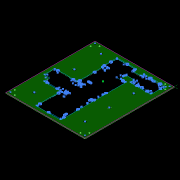
# Autodesk Inventor part: 3d_DAA_panel - Panel
Saved by Autodesk Inventor 2018 (Build 220112000, 112)
## iProperties
Created: 2024-08-29
Part Number: 3d_DAA_panel - Panel
Material: PCB
Document SubType Name: Modeling
Designer: cda1
Density: 4 g/cm^3
Appearance: PCB
Author: cda1
Autodesk Inventor part; units mm, degrees
(part 1 of 2)
ref_plane "YZ Plane" through (0, 0, 0) normal (1, 0, 0) x (0, 1, 0)
ref_plane "XZ Plane" through (0, 0, 0) normal (0, 1, 0) x (-1, 0, 0)
sketch "Boceto1" plane through (0, 0, 0) normal (0, 0, 1) x (1, 0, 0)
  circle A0 centre (-20.9021, 53.0601) radius 0.75 projected
  circle A1 centre (-25.9819, 53.0601) radius 0.75 projected
  circle A2 centre (-25.9819, 58.1399) radius 0.75 projected
  circle A3 centre (-23.442, 55.6) radius 0.7 projected
  circle A4 centre (-20.9021, 58.1399) radius 0.75 projected
  circle A5 centre (-9.192, 56.238) radius 1 projected
  circle A6 centre (-23.092, 32.962) radius 1 projected
  arc A7 (-27.742, 29.842) -> (-27.242, 29.342) centre (-27.242, 29.842) ccw projected
  line L0 (-27.242, 29.342) -> (-20.642, 29.342) projected
  arc A8 (-20.642, 29.342) -> (-20.142, 29.842) centre (-20.642, 29.842) ccw projected
  line L1 (-20.142, 29.842) -> (-20.142, 31.9) projected
  arc A9 (-19.642, 32.4) -> (-20.142, 31.9) centre (-19.642, 31.9) ccw projected
  line L2 (-19.642, 32.4) -> (12.558, 32.4) projected
  arc A10 (12.558, 32.4) -> (13.058, 32.9) centre (12.558, 32.9) ccw projected
  line L3 (13.058, 32.9) -> (13.058, 59.358) projected
  arc A11 (13.058, 59.358) -> (12.558, 59.858) centre (12.558, 59.358) ccw projected
  line L4 (12.558, 59.858) -> (-27.242, 59.858) projected
  arc A12 (-27.242, 59.858) -> (-27.742, 59.358) centre (-27.242, 59.358) ccw projected
  line L5 (-27.742, 29.842) -> (-27.742, 59.358) projected
  circle A13 centre (56.15, 55.6) radius 2 projected
  circle A14 centre (56.15, 33.6) radius 2 projected
  circle A15 centre (73, 53.6) radius 1.5 projected
  circle A16 centre (44.6, 53.6) radius 1.5 projected
  circle A17 centre (44.6, 35.6) radius 1.5 projected
  circle A18 centre (73, 35.6) radius 1.5 projected
  circle A19 centre (36.4, 32.98) radius 1 projected
  circle A20 centre (78.021, 53.178) radius 1 projected
  circle A21 centre (36.4, 56.256) radius 1 projected
  arc A22 (76.8, 32.3) -> (77.3, 32.8) centre (76.8, 32.8) ccw projected
  line L6 (77.3, 32.8) -> (77.3, 50.2) projected
  arc A23 (77.8, 50.7) -> (77.3, 50.2) centre (77.8, 50.2) ccw projected
  line L7 (77.8, 50.7) -> (79.8, 50.7) projected
  arc A24 (79.8, 50.7) -> (80.3, 51.2) centre (79.8, 51.2) ccw projected
  line L8 (80.3, 51.2) -> (80.3, 56.4) projected
  arc A25 (80.3, 56.4) -> (79.8, 56.9) centre (79.8, 56.4) ccw projected
  line L9 (79.8, 56.9) -> (58.9, 56.9) projected
  arc A26 (58.4, 57.4) -> (58.9, 56.9) centre (58.9, 57.4) ccw projected
  arc A27 (58.4, 57.4) -> (57.9, 57.9) centre (57.9, 57.4) ccw projected
  line L10 (57.9, 57.9) -> (54.4, 57.9) projected
  arc A28 (54.4, 57.9) -> (53.9, 57.4) centre (54.4, 57.4) ccw projected
  arc A29 (53.4, 56.9) -> (53.9, 57.4) centre (53.4, 57.4) ccw projected
  line L11 (53.4, 56.9) -> (39.4, 56.9) projected
  arc A30 (38.9, 57.4) -> (39.4, 56.9) centre (39.4, 57.4) ccw projected
  line L12 (38.9, 57.4) -> (38.9, 58.3) projected
  arc A31 (38.9, 58.3) -> (38.4, 58.8) centre (38.4, 58.3) ccw projected
  line L13 (38.4, 58.8) -> (34.4, 58.8) projected
  arc A32 (34.4, 58.8) -> (33.9, 58.3) centre (34.4, 58.3) ccw projected
  line L14 (33.9, 58.3) -> (33.9, 54.2) projected
  arc A33 (33.9, 54.2) -> (34.4, 53.7) centre (34.4, 54.2) ccw projected
  line L15 (34.4, 53.7) -> (36.8, 53.7) projected
  arc A34 (37.3, 53.2) -> (36.8, 53.7) centre (36.8, 53.2) ccw projected
  line L16 (37.3, 53.2) -> (37.3, 36) projected
  arc A35 (36.8, 35.5) -> (37.3, 36) centre (36.8, 36) ccw projected
  line L17 (36.8, 35.5) -> (34.4, 35.5) projected
  arc A36 (34.4, 35.5) -> (33.9, 35) centre (34.4, 35) ccw projected
  line L18 (33.9, 30.9) -> (33.9, 35) projected
  arc A37 (33.9, 30.9) -> (34.4, 30.4) centre (34.4, 30.9) ccw projected
  line L19 (34.4, 30.4) -> (38.4, 30.4) projected
  arc A38 (38.4, 30.4) -> (38.9, 30.9) centre (38.4, 30.9) ccw projected
  line L20 (38.9, 30.9) -> (38.9, 31.8) projected
  arc A39 (39.4, 32.3) -> (38.9, 31.8) centre (39.4, 31.8) ccw projected
  line L21 (39.4, 32.3) -> (53.4, 32.3) projected
  arc A40 (53.9, 31.8) -> (53.4, 32.3) centre (53.4, 31.8) ccw projected
  arc A41 (53.9, 31.8) -> (54.4, 31.3) centre (54.4, 31.8) ccw projected
  line L22 (54.4, 31.3) -> (57.9, 31.3) projected
  arc A42 (57.9, 31.3) -> (58.4, 31.8) centre (57.9, 31.8) ccw projected
  arc A43 (58.9, 32.3) -> (58.4, 31.8) centre (58.9, 31.8) ccw projected
  line L23 (58.9, 32.3) -> (76.8, 32.3) projected
  circle A44 centre (-9.825, -17.035) radius 0.37 projected
  circle A45 centre (-9.825, -15.765) radius 0.37 projected
  circle A46 centre (-11.095, -17.035) radius 0.37 projected
  circle A47 centre (-12.365, -17.035) radius 0.37 projected
  circle A48 centre (-13.635, -17.035) radius 0.37 projected
  circle A49 centre (-14.905, -15.765) radius 0.37 projected
  circle A50 centre (-16.175, -17.035) radius 0.37 projected
  circle A51 centre (-16.175, -15.765) radius 0.37 projected
  circle A52 centre (-14.905, -17.035) radius 0.37 projected
  circle A53 centre (-13.635, -15.765) radius 0.37 projected
  circle A54 centre (-12.365, -15.765) radius 0.37 projected
  circle A55 centre (-11.095, -15.765) radius 0.37 projected
  arc A56 (-20.107, 25.5) -> (-20.607, 26) centre (-20.607, 25.5) ccw projected
  line L24 (-25.5, 26) -> (-20.607, 26) projected
  arc A57 (-25.5, 26) -> (-26, 25.5) centre (-25.5, 25.5) ccw projected
  line L25 (-26, -28) -> (-26, 25.5) projected
  arc A58 (-26, -28) -> (-25.5, -28.5) centre (-25.5, -28) ccw projected
  line L26 (-16, -28.5) -> (-25.5, -28.5) projected
  arc A59 (-16, -28.5) -> (-15.5, -28) centre (-16, -28) ccw projected
  line L27 (-15.5, -26.5) -> (-15.5, -28) projected
  arc A60 (-15, -26) -> (-15.5, -26.5) centre (-15, -26.5) ccw projected
  line L28 (25.5, -26) -> (-15, -26) projected
  arc A61 (25.5, -26) -> (26, -25.5) centre (25.5, -25.5) ccw projected
  line L29 (26, 22) -> (26, -25.5) projected
  arc A62 (26, 22) -> (25, 23) centre (25, 22) ccw projected
  line L30 (25, 23) -> (-19.607, 23) projected
  arc A63 (-20.107, 23.5) -> (-19.607, 23) centre (-19.607, 23.5) ccw projected
  line L31 (-20.107, 23.5) -> (-20.107, 25.5) projected
  arc A64 (-15.5, -32.942) -> (-16, -32.442) centre (-16, -32.942) ccw projected
  line L32 (-16, -32.442) -> (-22.3, -32.442) projected
  arc A65 (-22.3, -32.442) -> (-22.8, -32.942) centre (-22.3, -32.942) ccw projected
  line L33 (-22.8, -32.942) -> (-22.8, -62.458) projected
  arc A66 (-22.8, -62.458) -> (-22.3, -62.958) centre (-22.3, -62.458) ccw projected
  line L34 (-22.3, -62.958) -> (-16, -62.958) projected
  arc A67 (-16, -62.958) -> (-15.5, -62.458) centre (-16, -62.458) ccw projected
  line L35 (-15.5, -62.458) -> (-15.5, -60.4) projected
  arc A68 (-15, -59.9) -> (-15.5, -60.4) centre (-15, -60.4) ccw projected
  line L36 (-15, -59.9) -> (25.5, -59.9) projected
  arc A69 (25.5, -59.9) -> (26, -59.4) centre (25.5, -59.4) ccw projected
  line L37 (26, -36) -> (26, -59.4) projected
  arc A70 (26, -36) -> (25.5, -35.5) centre (25.5, -36) ccw projected
  line L38 (25.5, -35.5) -> (-15, -35.5) projected
  arc A71 (-15.5, -35) -> (-15, -35.5) centre (-15, -35) ccw projected
  line L39 (-15.5, -35) -> (-15.5, -32.942) projected
  circle A72 centre (22.935, -52.24) radius 0.37 projected
  circle A73 centre (21.665, -52.24) radius 0.37 projected
  circle A74 centre (21.665, -50.97) radius 0.37 projected
  circle A75 centre (21.665, -49.7) radius 0.37 projected
  circle A76 centre (22.935, -48.43) radius 0.37 projected
  circle A77 centre (21.665, -47.16) radius 0.37 projected
  circle A78 centre (22.935, -47.16) radius 0.37 projected
  circle A79 centre (21.665, -48.43) radius 0.37 projected
  circle A80 centre (22.935, -49.7) radius 0.37 projected
  circle A81 centre (22.935, -50.97) radius 0.37 projected
  circle A82 centre (-19.1, -36.062) radius 1 projected
  circle A83 centre (-19.1, -59.338) radius 1 projected
  circle A84 centre (-47.178, -49.615) radius 0.65 projected
  circle A85 centre (-50.172, -48.173) radius 0.65 projected
  circle A86 centre (-48.1, -45.575) radius 0.65 projected
  circle A87 centre (-44.129, -48.182) radius 0.65 projected
  circle A88 centre (-46.241, -51.242) radius 0.65 projected
  circle A89 centre (-49.959, -51.242) radius 0.65 projected
  circle A90 centre (-52.071, -48.182) radius 0.65 projected
  circle A91 centre (-50.752, -44.706) radius 0.65 projected
  circle A92 centre (-47.143, -43.816) radius 0.65 projected
  circle A93 centre (-44.36, -46.282) radius 0.65 projected
  circle A94 centre (-42.297, -46.781) radius 0.65 projected
  circle A95 centre (-42.865, -50.367) radius 0.65 projected
  circle A96 centre (-45.433, -52.935) radius 0.65 projected
  circle A97 centre (-49.019, -53.503) radius 0.65 projected
  circle A98 centre (-52.254, -51.854) radius 0.65 projected
  circle A99 centre (-53.903, -48.619) radius 0.65 projected
  circle A100 centre (-53.335, -45.033) radius 0.65 projected
  circle A101 centre (-50.767, -42.465) radius 0.65 projected
  circle A102 centre (-47.181, -41.897) radius 0.65 projected
  circle A103 centre (-43.946, -43.546) radius 0.65 projected
  circle A104 centre (-41.884, -52.328) radius 0.65 projected
  circle A105 centre (-44.622, -54.626) radius 0.65 projected
  circle A106 centre (-48.1, -55.45) radius 0.65 projected
  circle A107 centre (-51.578, -54.626) radius 0.65 projected
  circle A108 centre (-54.316, -52.328) radius 0.65 projected
  circle A109 centre (-55.732, -49.046) radius 0.65 projected
  circle A110 centre (-55.524, -45.477) radius 0.65 projected
  circle A111 centre (-53.737, -42.382) radius 0.65 projected
  circle A112 centre (-50.751, -40.417) radius 0.65 projected
  circle A113 centre (-47.2, -40.002) radius 0.65 projected
  circle A114 centre (-43.841, -41.225) radius 0.65 projected
  circle A115 centre (-41.388, -43.825) radius 0.65 projected
  circle A116 centre (-40.363, -47.249) radius 0.65 projected
  circle A117 centre (-56.355, -55.955) radius 0.65 projected
  circle A118 centre (-48.1, -47.7) radius 0.65 projected
  circle A119 centre (-39.845, -39.445) radius 0.65 projected
  circle A120 centre (-56.355, -39.445) radius 0.65 projected
  circle A121 centre (-39.845, -55.955) radius 0.65 projected
  circle A122 centre (-40.468, -49.046) radius 0.65 projected
  circle A123 centre (-40.676, -45.477) radius 0.65 projected
  circle A124 centre (-42.463, -42.382) radius 0.65 projected
  circle A125 centre (-45.449, -40.417) radius 0.65 projected
  circle A126 centre (-49, -40.002) radius 0.65 projected
  circle A127 centre (-52.359, -41.225) radius 0.65 projected
  circle A128 centre (-54.812, -43.825) radius 0.65 projected
  circle A129 centre (-55.837, -47.249) radius 0.65 projected
  circle A130 centre (-55.216, -50.77) radius 0.65 projected
  circle A131 centre (-53.082, -53.637) radius 0.65 projected
  circle A132 centre (-49.887, -55.241) radius 0.65 projected
  circle A133 centre (-46.313, -55.241) radius 0.65 projected
  circle A134 centre (-43.118, -53.637) radius 0.65 projected
  circle A135 centre (-40.984, -50.77) radius 0.65 projected
  circle A136 centre (-45.433, -42.465) radius 0.65 projected
  circle A137 centre (-49.019, -41.897) radius 0.65 projected
  circle A138 centre (-52.254, -43.546) radius 0.65 projected
  circle A139 centre (-53.903, -46.781) radius 0.65 projected
  circle A140 centre (-53.335, -50.367) radius 0.65 projected
  circle A141 centre (-50.767, -52.935) radius 0.65 projected
  circle A142 centre (-47.181, -53.503) radius 0.65 projected
  circle A143 centre (-43.946, -51.854) radius 0.65 projected
  circle A144 centre (-42.297, -48.619) radius 0.65 projected
  circle A145 centre (-42.865, -45.033) radius 0.65 projected
  circle A146 centre (-45.448, -44.706) radius 0.65 projected
  circle A147 centre (-49.057, -43.816) radius 0.65 projected
  circle A148 centre (-51.84, -46.282) radius 0.65 projected
  circle A149 centre (-51.392, -49.972) radius 0.65 projected
  circle A150 centre (-48.1, -51.7) radius 0.65 projected
  circle A151 centre (-44.808, -49.972) radius 0.65 projected
  circle A152 centre (-46.439, -46.375) radius 0.65 projected
  circle A153 centre (-49.761, -46.375) radius 0.65 projected
  circle A154 centre (-49.022, -49.615) radius 0.65 projected
  circle A155 centre (-46.028, -48.173) radius 0.65 projected
  arc A156 (-77.3, -49.2) -> (-75.3, -51.2) centre (-75.3, -49.2) ccw projected
  line L40 (-75.3, -51.2) -> (-71.048, -51.2) projected
  arc A157 (-65.048, -57.2) -> (-71.048, -51.2) centre (-71.048, -57.2) ccw projected
  line L41 (-65.048, -57.2) -> (-65.048, -62.7) projected
  arc A158 (-65.048, -62.7) -> (-63.048, -64.7) centre (-63.048, -62.7) ccw projected
  line L42 (-30.8, -64.7) -> (-63.048, -64.7) projected
  arc A159 (-30.8, -64.7) -> (-30.3, -64.2) centre (-30.8, -64.2) ccw projected
  line L43 (-30.3, -64.2) -> (-30.3, -31.2) projected
  arc A160 (-30.3, -31.2) -> (-30.8, -30.7) centre (-30.8, -31.2) ccw projected
  line L44 (-76.8, -30.7) -> (-30.8, -30.7) projected
  arc A161 (-76.8, -30.7) -> (-77.3, -31.2) centre (-76.8, -31.2) ccw projected
  line L45 (-77.3, -31.2) -> (-77.3, -49.2) projected
  circle A162 centre (-67.2, -34.022) radius 1 projected
  circle A163 centre (-36.6, -34.022) radius 1 projected
  circle A164 centre (-36.6, -61.378) radius 1 projected
  arc A165 (-25.5, -66.1) -> (-26, -66.6) centre (-25.5, -66.6) ccw projected
  line L46 (-26, -120.1) -> (-26, -66.6) projected
  arc A166 (-26, -120.1) -> (-25.5, -120.6) centre (-25.5, -120.1) ccw projected
  line L47 (25.5, -120.6) -> (-25.5, -120.6) projected
  arc A167 (25.5, -120.6) -> (26, -120.1) centre (25.5, -120.1) ccw projected
  line L48 (26, -73.9) -> (26, -120.1) projected
  arc A168 (26, -73.9) -> (25.5, -73.4) centre (25.5, -73.9) ccw projected
  line L49 (25.5, -73.4) -> (-15, -73.4) projected
  arc A169 (-15.5, -72.9) -> (-15, -73.4) centre (-15, -72.9) ccw projected
  line L50 (-15.5, -72.9) -> (-15.5, -66.6) projected
  arc A170 (-15.5, -66.6) -> (-16, -66.1) centre (-16, -66.6) ccw projected
  line L51 (-25.5, -66.1) -> (-16, -66.1) projected
  circle A171 centre (23.035, -108.94) radius 0.37 projected
  circle A172 centre (21.765, -108.94) radius 0.37 projected
  circle A173 centre (21.765, -107.67) radius 0.37 projected
  circle A174 centre (21.765, -106.4) radius 0.37 projected
  circle A175 centre (21.765, -105.13) radius 0.37 projected
  circle A176 centre (23.035, -103.86) radius 0.37 projected
  circle A177 centre (21.765, -103.86) radius 0.37 projected
  circle A178 centre (23.035, -105.13) radius 0.37 projected
  circle A179 centre (23.035, -106.4) radius 0.37 projected
  circle A180 centre (23.035, -107.67) radius 0.37 projected
  line L52 (-87.3, 69.858) -> (90.3, 69.858)
  line L53 (90.3, 69.858) -> (90.3, -130.6)
  line L54 (90.3, -130.6) -> (-87.3, -130.6)
  line L55 (-87.3, -130.6) -> (-87.3, 69.858)
  line L56 (14.1664, 40.6) -> (14.1664, 52) projected
  line L57 (14.1664, 52) -> (13.0584, 52) projected
  line L58 (13.0584, 40.6) -> (13.0584, 52) projected
  line L59 (14.1664, 40.6) -> (13.0584, 40.6) projected
  line L60 (14.1664, 40.6) -> (14.1664, 52) projected
  line L61 (18.9048, 40.6) -> (14.1664, 40.6) projected
  line L62 (18.9048, 40.6) -> (18.9048, 52) projected
  line L63 (18.9048, 52) -> (14.1664, 52) projected
  line L64 (18.9048, 40.6) -> (18.9048, 52) projected
  line L65 (27.24, 40.6) -> (18.9048, 40.6) projected
  line L66 (27.24, 40.6) -> (27.24, 52) projected
  line L67 (27.24, 52) -> (18.9048, 52) projected
  line L68 (27.24, 40.6) -> (27.24, 52) projected
  line L69 (36.2006, 40.6) -> (27.24, 40.6) projected
  line L70 (36.2006, 40.6) -> (36.2006, 52) projected
  line L71 (36.2006, 52) -> (27.24, 52) projected
  line L72 (36.2006, 40.6) -> (36.2006, 52) projected
  line L73 (37.3, 40.6) -> (36.2006, 40.6) projected
  line L74 (37.3, 40.6) -> (37.3, 52) projected
  line L75 (37.3, 52) -> (36.2006, 52) projected
  line L76 (-17.807, 32.1945) -> (7.393, 32.1945) projected
  line L77 (7.393, 32.4003) -> (7.393, 32.1945) projected
  line L78 (-17.807, 32.4003) -> (7.393, 32.4003) projected
  line L79 (-17.807, 32.1945) -> (-17.807, 32.4003) projected
  line L80 (-17.807, 32.1945) -> (7.393, 32.1945) projected
  line L81 (-17.807, 30.0192) -> (-17.807, 32.1945) projected
  line L82 (-17.807, 30.0192) -> (7.393, 30.0192) projected
  line L83 (7.393, 32.1945) -> (7.393, 30.0192) projected
  line L84 (-17.807, 30.0192) -> (7.393, 30.0192) projected
  line L85 (-17.807, 24.6786) -> (-17.807, 30.0192) projected
  line L86 (-17.807, 24.6786) -> (7.393, 24.6786) projected
  line L87 (7.393, 30.0192) -> (7.393, 24.6786) projected
  line L88 (-17.807, 24.3258) -> (7.393, 24.3258) projected
  line L89 (-17.807, 23.636) -> (-17.807, 24.3258) projected
  line L90 (-17.807, 23.636) -> (7.393, 23.636) projected
  line L91 (7.393, 24.3258) -> (7.393, 23.636) projected
  line L92 (-17.807, 24.6786) -> (7.393, 24.6786) projected
  line L93 (-17.807, 24.3258) -> (-17.807, 24.6786) projected
  line L94 (-17.807, 24.3258) -> (7.393, 24.3258) projected
  line L95 (7.393, 24.6786) -> (7.393, 24.3258) projected
  line L96 (-17.807, 23.636) -> (7.393, 23.636) projected
  line L97 (-17.807, 23) -> (-17.807, 23.636) projected
  line L98 (7.393, 23) -> (-17.807, 23) projected
  line L99 (7.393, 23.636) -> (7.393, 23) projected
  line L100 (24.5, -26.636) -> (-13, -26.636) projected
  line L101 (24.5, -26) -> (24.5, -26.636) projected
  line L102 (-13, -26) -> (24.5, -26) projected
  line L103 (-13, -26.636) -> (-13, -26) projected
  line L104 (24.5, -27.3258) -> (-13, -27.3258) projected
  line L105 (24.5, -26.636) -> (24.5, -27.3258) projected
  line L106 (24.5, -26.636) -> (-13, -26.636) projected
  line L107 (-13, -27.3258) -> (-13, -26.636) projected
  line L108 (24.5, -27.6786) -> (-13, -27.6786) projected
  line L109 (24.5, -27.3258) -> (24.5, -27.6786) projected
  line L110 (24.5, -27.3258) -> (-13, -27.3258) projected
  line L111 (-13, -27.6786) -> (-13, -27.3258) projected
  line L112 (24.5, -33.0192) -> (-13, -33.0192) projected
  line L113 (24.5, -27.6786) -> (24.5, -33.0192) projected
  line L114 (24.5, -27.6786) -> (-13, -27.6786) projected
  line L115 (-13, -33.0192) -> (-13, -27.6786) projected
  line L116 (24.5, -35.1945) -> (-13, -35.1945) projected
  line L117 (24.5, -33.0192) -> (24.5, -35.1945) projected
  line L118 (24.5, -33.0192) -> (-13, -33.0192) projected
  line L119 (-13, -35.1945) -> (-13, -33.0192) projected
  line L120 (24.5, -35.1945) -> (-13, -35.1945) projected
  line L121 (-13, -35.5003) -> (-13, -35.1945) projected
  line L122 (24.5, -35.5003) -> (-13, -35.5003) projected
  line L123 (24.5, -35.1945) -> (24.5, -35.5003) projected
  line L124 (-24.064, -38) -> (-24.064, -59.3) projected
  line L125 (-24.064, -59.3) -> (-22.8, -59.3) projected
  line L126 (-22.8, -38) -> (-22.8, -59.3) projected
  line L127 (-24.064, -38) -> (-22.8, -38) projected
  line L128 (-24.064, -38) -> (-24.064, -59.3) projected
  line L129 (-28.2863, -38) -> (-24.064, -38) projected
  line L130 (-28.2863, -38) -> (-28.2863, -59.3) projected
  line L131 (-28.2863, -59.3) -> (-24.064, -59.3) projected
  line L132 (-28.2863, -38) -> (-28.2863, -59.3) projected
  line L133 (-30.2998, -38) -> (-28.2863, -38) projected
  line L134 (-30.2998, -38) -> (-30.2998, -59.3) projected
  line L135 (-30.2998, -59.3) -> (-28.2863, -59.3) projected
  line L136 (24.5, -72.6558) -> (-13, -72.6558) projected
  line L137 (-13, -72.6558) -> (-13, -73.4) projected
  line L138 (24.5, -73.4) -> (-13, -73.4) projected
  line L139 (24.5, -72.6558) -> (24.5, -73.4) projected
  line L140 (24.5, -72.6558) -> (-13, -72.6558) projected
  line L141 (24.5, -71.0155) -> (24.5, -72.6558) projected
  line L142 (24.5, -71.0155) -> (-13, -71.0155) projected
  line L143 (-13, -71.0155) -> (-13, -72.6558) projected
  line L144 (24.5, -71.0155) -> (-13, -71.0155) projected
  line L145 (24.5, -61.4174) -> (24.5, -71.0155) projected
  line L146 (24.5, -61.4174) -> (-13, -61.4174) projected
  line L147 (-13, -61.4174) -> (-13, -71.0155) projected
  line L148 (24.5, -61.4174) -> (-13, -61.4174) projected
  line L149 (24.5, -61.3135) -> (24.5, -61.4174) projected
  line L150 (24.5, -61.3135) -> (-13, -61.3135) projected
  line L151 (-13, -61.3135) -> (-13, -61.4174) projected
  line L152 (24.5, -61.3135) -> (-13, -61.3135) projected
  line L153 (24.5, -60.0991) -> (24.5, -61.3135) projected
  line L154 (24.5, -60.0991) -> (-13, -60.0991) projected
  line L155 (-13, -60.0991) -> (-13, -61.3135) projected
  line L156 (24.5, -60.0991) -> (-13, -60.0991) projected
  line L157 (24.5, -59.8978) -> (24.5, -60.0991) projected
  line L158 (24.5, -59.8978) -> (-13, -59.8978) projected
  line L159 (-13, -59.8978) -> (-13, -60.0991) projected
  line L160 (-79.3, -29.7) -> (-79.3, -52.2)
  arc A181 (-67.048, -57.2) -> (-71.048, -53.2) centre (-71.048, -57.2) ccw
  line L161 (-71.048, -53.2) -> (-78.3, -53.2)
  line L162 (-67.048, -57.2) -> (-67.048, -65.7)
  line L163 (15.058, 25) -> (15.058, 34.6)
  line L164 (15.058, 36.6) -> (31.9, 36.6)
  line L165 (31.9, 36.6) -> (31.9, 29.4)
  line L166 (79.3, 29.4) -> (79.3, 47.7)
  line L167 (80.3, 48.7) -> (81.3, 48.7)
  line L168 (82.3, 49.7) -> (82.3, 59.8)
  line L169 (31.9, 59.8) -> (31.9, 56)
  line L170 (31.9, 56) -> (15.058, 56)
  line L171 (15.058, 58) -> (15.058, 60.858)
  line L172 (-28.742, 27.342) -> (-28, 27.342)
  arc A182 (-78.3, -28.7) -> (-79.3, -29.7) centre (-78.3, -29.7) ccw
  arc A183 (-79.3, -52.2) -> (-78.3, -53.2) centre (-78.3, -52.2) ccw
  arc A184 (-67.048, -65.7) -> (-66.048, -66.7) centre (-66.048, -65.7) ccw
  arc A185 (-28, -121.6) -> (-27, -122.6) centre (-27, -121.6) ccw
  arc A186 (27, -122.6) -> (28, -121.6) centre (27, -121.6) ccw
  arc A187 (28, 24) -> (27, 25) centre (27, 24) ccw
  arc A188 (31.9, 29.4) -> (32.9, 28.4) centre (32.9, 29.4) ccw
  arc A189 (78.3, 28.4) -> (79.3, 29.4) centre (78.3, 29.4) ccw
  arc A190 (80.3, 48.7) -> (79.3, 47.7) centre (80.3, 47.7) ccw
  arc A191 (81.3, 48.7) -> (82.3, 49.7) centre (81.3, 49.7) ccw
  arc A192 (82.3, 59.8) -> (81.3, 60.8) centre (81.3, 59.8) ccw
  arc A193 (32.9, 60.8) -> (31.9, 59.8) centre (32.9, 59.8) ccw
  arc A194 (15.058, 60.858) -> (14.058, 61.858) centre (14.058, 60.858) ccw
  arc A195 (-28.742, 61.858) -> (-29.742, 60.858) centre (-28.742, 60.858) ccw
  arc A196 (-29.742, 28.342) -> (-28.742, 27.342) centre (-28.742, 28.342) ccw
  line L173 (-20.3, -28.5) -> (-18.3, -28.5)
  line L174 (-18.3, -28.5) -> (-18.3, -32.442)
  line L175 (-18.3, -32.442) -> (-20.3, -32.442)
  line L176 (-20.3, -32.442) -> (-20.3, -28.5)
  line L177 (-20.3, -62.958) -> (-18.3, -62.958)
  line L178 (-18.3, -62.958) -> (-18.3, -66.1)
  line L179 (-18.3, -66.1) -> (-20.3, -66.1)
  line L180 (-20.3, -66.1) -> (-20.3, -62.958)
  line L181 (-60.048, -64.7) -> (-60.048, -66.7)
  line L182 (-58.048, -64.7) -> (-58.048, -66.7)
  line L183 (-37.3, -64.7) -> (-37.3, -66.7)
  line L184 (-35.3, -64.7) -> (-35.3, -66.7)
  line L185 (-72.3, -28.7) -> (-72.3, -30.7)
  line L186 (-70.3, -28.7) -> (-70.3, -30.7)
  line L187 (-37.3, -28.7) -> (-37.3, -30.7)
  line L188 (-35.3, -28.7) -> (-35.3, -30.7)
  line L189 (-29.742, 31.342) -> (-27.742, 31.342)
  line L190 (-29.742, 33.342) -> (-27.742, 33.342)
  line L191 (-29.742, 47.858) -> (-27.742, 47.858)
  line L192 (-27.742, 45.858) -> (-29.742, 45.858)
  line L193 (15.058, 36.6) -> (13.058, 36.6)
  line L194 (15.058, 34.6) -> (13.058, 34.6)
  line L195 (15.058, 56) -> (13.058, 56)
  line L196 (15.058, 58) -> (13.058, 58)
  line L197 (48.7, 56.9) -> (48.7, 60.8)
  line L198 (46.7, 56.9) -> (46.7, 60.8)
  line L199 (68.7, 56.9) -> (68.7, 60.8)
  line L200 (70.7, 56.9) -> (70.7, 60.8)
  line L201 (70.7, 32.3) -> (70.7, 28.4)
  line L202 (68.7, 32.3) -> (68.7, 28.4)
  line L203 (48.7, 32.3) -> (48.7, 28.4)
  line L204 (46.7, 32.3) -> (46.7, 28.4)
  line L205 (20, 25) -> (20, 23)
  line L206 (22, 25) -> (22, 23)
  line L207 (-26, 9.6) -> (-28, 9.6)
  line L208 (-26, 7.6) -> (-28, 7.6)
  line L209 (-26, -25.5) -> (-28, -25.5)
  line L210 (-26, -23.5) -> (-28, -23.5)
  line L211 (26, -21) -> (28, -21)
  line L212 (26, -19) -> (28, -19)
  line L213 (26, -45.7) -> (28, -45.7)
  line L214 (26, -49.7) -> (28, -49.7)
  line L215 (-28, -71.1) -> (-26, -71.1)
  line L216 (-28, -73.1) -> (-26, -73.1)
  line L217 (-28, -115.6) -> (-26, -115.6)
  line L218 (-28, -113.6) -> (-26, -113.6)
  line L219 (-1, -120.6) -> (-1, -122.6)
  line L220 (1, -120.6) -> (1, -122.6)
  line L221 (26, -81.8) -> (28, -81.8)
  line L222 (26, -83.8) -> (28, -83.8)
  line L223 (26, -113.6) -> (28, -113.6)
  line L224 (26, -115.6) -> (28, -115.6)
  line L225 (20, 23) -> (22, 23)
  line L226 (13.058, 34.6) -> (13.058, 36.6)
  line L227 (46.7, 32.3) -> (48.7, 32.3)
  line L228 (68.7, 32.3) -> (70.7, 32.3)
  line L229 (68.7, 56.9) -> (70.7, 56.9)
  line L230 (48.7, 56.9) -> (46.7, 56.9)
  line L231 (13.058, 58) -> (13.058, 56)
  line L232 (-27.742, 47.858) -> (-27.742, 45.858)
  line L233 (-27.742, 33.342) -> (-27.742, 31.342)
  line L234 (-26, 9.6) -> (-26, 7.6)
  line L235 (-26, -23.5) -> (-26, -25.5)
  line L236 (-35.3, -30.7) -> (-37.3, -30.7)
  line L237 (-72.3, -30.7) -> (-70.3, -30.7)
  line L238 (-60.048, -64.7) -> (-58.048, -64.7)
  line L239 (-37.3, -64.7) -> (-35.3, -64.7)
  line L240 (-26, -71.1) -> (-26, -73.1)
  line L241 (-26, -113.6) -> (-26, -115.6)
  line L242 (-1, -120.6) -> (1, -120.6)
  line L243 (26, -115.6) -> (26, -113.6)
  line L244 (26, -81.8) -> (26, -83.8)
  line L245 (26, -45.7) -> (26, -49.7)
  line L246 (26, -19) -> (26, -21)
  line L247 (-72.3, -28.7) -> (-78.3, -28.7)
  line L248 (-28, -28.7) -> (-35.3, -28.7)
  line L249 (-37.3, -28.7) -> (-70.3, -28.7)
  line L250 (-66.048, -66.7) -> (-60.048, -66.7)
  line L251 (-58.048, -66.7) -> (-37.3, -66.7)
  line L252 (-35.3, -66.7) -> (-28, -66.7)
  line L253 (-28, -66.7) -> (-28, -71.1)
  line L254 (-28, -73.1) -> (-28, -113.6)
  line L255 (-28, -115.6) -> (-28, -121.6)
  line L256 (-27, -122.6) -> (-1, -122.6)
  line L257 (1, -122.6) -> (27, -122.6)
  line L258 (28, -121.6) -> (28, -115.6)
  line L259 (28, -113.6) -> (28, -83.8)
  line L260 (28, -81.8) -> (28, -49.7)
  line L261 (28, -45.7) -> (28, -21)
  line L262 (28, -19) -> (28, 24)
  line L263 (27, 25) -> (22, 25)
  line L264 (20, 25) -> (15.058, 25)
  line L265 (32.9, 28.4) -> (46.7, 28.4)
  line L266 (48.7, 28.4) -> (68.7, 28.4)
  line L267 (70.7, 28.4) -> (78.3, 28.4)
  line L268 (81.3, 60.8) -> (70.7, 60.8)
  line L269 (68.7, 60.8) -> (48.7, 60.8)
  line L270 (46.7, 60.8) -> (32.9, 60.8)
  line L271 (-29.742, 60.858) -> (-29.742, 47.858)
  line L272 (-29.742, 45.858) -> (-29.742, 33.342)
  line L273 (-29.742, 31.342) -> (-29.742, 28.342)
  line L274 (-28, 27.342) -> (-28, 9.6)
  line L275 (-28, 7.6) -> (-28, -23.5)
  line L276 (-28, -25.5) -> (-28, -28.7)
  line L277 (26, -47.7) -> (28, -47.7) construction
  line L278 (-6.6, 61.858) -> (-6.6, 59.858)
  line L279 (-4.6, 61.858) -> (-4.6, 59.858)
  line L280 (-4.6, 59.858) -> (-6.6, 59.858)
  line L281 (14.058, 61.858) -> (-4.6, 61.858)
  line L282 (-6.6, 61.858) -> (-28.742, 61.858)
  point P0 (0, 0)
  dimension "d0" = 10
  dimension "d1" = 10
  dimension "d2" = 10
  dimension "d3" = 10
  dimension "d4" = 2
  dimension "d6" = 2
  dimension "d10" = 2
  dimension "d11" = 2
  dimension "d12" = 2
  dimension "d14" = 2
  dimension "d19" = 2
  dimension "d21" = 4
  dimension "d22" = 4
  dimension "d23" = 2
  dimension "d24" = 2
  dimension "d25" = 2
  dimension "d28" = 1
  dimension "d29" = 1
  dimension "d30" = 2
  dimension "d31" = 2
  dimension "d32" = 2.5
  dimension "d33" = 2
  dimension "d34" = 2
  dimension "d35" = 2
  dimension "d36" = 2
  dimension "d37" = 2
  dimension "d38" = 2
  dimension "d39" = 2
  dimension "d40" = 2
  dimension "d42" = 2
  dimension "d43" = 2
  dimension "d44" = 2
  dimension "d45" = 2
  dimension "d46" = 6.6
  dimension "d47" = 12.8
  dimension "d48" = 12.8
  dimension "d49" = 9.6
  dimension "d50" = 2
  dimension "d51" = 12
  dimension "d52" = 5
  dimension "d53" = 5
  dimension "d54" = 5
  dimension "d55" = 5
  dimension "d56" = 2
  dimension "d57" = 4
  dimension "d58" = 2
  dimension "d59" = 16.4
  dimension "d60" = 2
  dimension "d62" = 3
  dimension "d63" = 2
  dimension "d64" = 5
  dimension "d65" = 4
  dimension "d69" = 2
  dimension "d70" = 2
  dimension "d71" = 2
  dimension "d72" = 2
  dimension "d73" = 2
  dimension "d74" = 5
  dimension "d75" = 5
  dimension "d76" = 5
  dimension "d77" = 8.4
  dimension "d79" = 2
  dimension "d80" = 2
  dimension "d81" = 2
  constraints: 254 end point, 170 perpendicular, 63 tangent, 51 point on line, 32 point on circle, 18 collinear, 16 centre point, 16 parallel, 13 equal radius, 11 horizontal, 3 vertical, 1 coincident, 1 midpoint, 1 vertical alignment
  measures "d0" distance between parallel lines of L54 L47
  measures "d1" distance between parallel lines of L52 L4
  measures "d2" distance between parallel lines of L55 L45
  measures "d3" distance between parallel lines of L53 L8
  measures "d4" distance between parallel lines of L162 L41
  measures "d6" distance between parallel lines of L160 L45
  measures "d10" distance between parallel lines of L0 L172
  measures "d11" distance between parallel lines of L163 L3
  measures "d12" distance between parallel lines of L171 L3
  measures "d14" distance between parallel lines of L165 L18
  measures "d19" distance between parallel lines of L14 L169
  measures "d21" distance between parallel lines of L67 L170
  measures "d22" distance between parallel lines of L164 L65
  measures "d23" distance between parallel lines of L166 L6
  measures "d24" distance between parallel lines of L168 L8
  measures "d25" distance between parallel lines of L167 L7
  measures "d28" radius of A182
  measures "d29" radius of A189
  measures "d30" distance between parallel lines of L176 L174
  measures "d31" distance between parallel lines of L178 L180
  measures "d32" distance between parallel lines of L33 L176
  measures "d33" distance between parallel lines of L182 L181
  measures "d34" distance between parallel lines of L184 L183
  measures "d35" distance between parallel lines of L185 L186
  measures "d36" distance between parallel lines of L187 L188
  measures "d37" distance between parallel lines of L189 L190
  measures "d38" distance between parallel lines of L191 L192
  measures "d39" distance between parallel lines of L194 L193
  measures "d40" distance between parallel lines of L195 L196
  measures "d42" distance between parallel lines of L198 L197
  measures "d43" distance between parallel lines of L204 L203
  measures "d44" distance between parallel lines of L202 L201
  measures "d45" distance between parallel lines of L200 L199
  measures "d46" distance between parallel lines of L6 L201
  measures "d47" distance between parallel lines of L18 L204
  measures "d48" distance between parallel lines of L14 L198
  measures "d49" distance between parallel lines of L8 L200
  measures "d50" distance between parallel lines of L0 L189
  measures "d51" distance between parallel lines of L4 L191
  measures "d52" distance from line of L185 L45.start
  measures "d53" distance from line of L188 L43.end
  measures "d54" distance from line of L184 L43.start
  measures "d55" distance from line of L41.end L181
  measures "d56" distance between parallel lines of L206 L205
  measures "d57" distance between parallel lines of L206 L29
  measures "d58" distance between parallel lines of L208 L207
  measures "d59" distance between parallel lines of L24 L207
  measures "d60" distance between parallel lines of L209 L210
  measures "d62" distance from line of L209 L26.end
  measures "d63" distance between parallel lines of L211 L212
  measures "d64" distance between parallel lines of L211 L28
  measures "d65" distance between parallel lines of L213 L214
  measures "d69" distance between parallel lines of L224 L223
  measures "d70" distance between parallel lines of L222 L221
  measures "d71" distance between parallel lines of L220 L219
  measures "d72" distance between parallel lines of L218 L217
  measures "d73" distance between parallel lines of L216 L215
  measures "d74" distance between parallel lines of L51 L215
  measures "d75" distance between parallel lines of L47 L217
  measures "d76" distance between parallel lines of L47 L224
  measures "d77" distance between parallel lines of L49 L221
  measures "d79" distance from line of L247 L44.start
  measures "d80" distance from line of L42.end L250
  measures "d81" distance between parallel lines of L46 L253
extrude "Extrusión1" add sketch "Boceto1" against normal blind 1.742 contours L26 L174 L32 L176 | L34 L178 L51 L180 | L52 L53 L54 L55
sketch "Boceto2" plane through (0, 0, 0) normal (0, 0, 1) x (1, 0, 0)
  line L0 (-26, 7.6) -> (-26, 9.6) construction
  line L1 (-26, 9.6) -> (-28, 9.6) construction
  line L2 (-28, 9.6) -> (-28, 27.342) construction
  line L3 (-28, 27.342) -> (-28.742, 27.342) construction
  arc A0 (-29.742, 28.342) -> (-28.742, 27.342) centre (-28.742, 28.342) ccw construction
  line L4 (-29.742, 28.342) -> (-29.742, 31.342) construction
  line L5 (-29.742, 31.342) -> (-27.742, 31.342) construction
  line L6 (-27.742, 31.342) -> (-27.742, 33.342) construction
  line L7 (-27.742, 33.342) -> (-29.742, 33.342) construction
  line L8 (-29.742, 33.342) -> (-29.742, 45.858) construction
  line L9 (-29.742, 45.858) -> (-27.742, 45.858) construction
  line L10 (-27.742, 45.858) -> (-27.742, 47.858) construction
  line L11 (-27.742, 47.858) -> (-29.742, 47.858) construction
  line L12 (-29.742, 47.858) -> (-29.742, 60.858) construction
  arc A1 (-28.742, 61.858) -> (-29.742, 60.858) centre (-28.742, 60.858) ccw construction
  line L13 (-4.6, 61.858) -> (14.058, 61.858) construction
  arc A2 (15.058, 60.858) -> (14.058, 61.858) centre (14.058, 60.858) ccw construction
  line L14 (15.058, 60.858) -> (15.058, 58) construction
  line L15 (15.058, 58) -> (13.058, 58) construction
  line L16 (13.058, 36.6) -> (13.058, 34.6) construction
  line L17 (13.058, 56) -> (31.9, 56) construction
  line L18 (31.9, 56) -> (31.9, 59.8) construction
  arc A3 (32.9, 60.8) -> (31.9, 59.8) centre (32.9, 59.8) ccw construction
  line L19 (32.9, 60.8) -> (46.7, 60.8) construction
  line L20 (46.7, 60.8) -> (46.7, 56.9) construction
  line L21 (46.7, 56.9) -> (48.7, 56.9) construction
  line L22 (48.7, 56.9) -> (48.7, 60.8) construction
  line L23 (48.7, 60.8) -> (68.7, 60.8) construction
  line L24 (68.7, 60.8) -> (68.7, 56.9) construction
  line L25 (68.7, 56.9) -> (70.7, 56.9) construction
  line L26 (70.7, 56.9) -> (70.7, 60.8) construction
  line L27 (70.7, 60.8) -> (81.3, 60.8) construction
  arc A4 (82.3, 59.8) -> (81.3, 60.8) centre (81.3, 59.8) ccw construction
  line L28 (82.3, 59.8) -> (82.3, 49.7) construction
  arc A5 (81.3, 48.7) -> (82.3, 49.7) centre (81.3, 49.7) ccw construction
  line L29 (81.3, 48.7) -> (80.3, 48.7) construction
  arc A6 (80.3, 48.7) -> (79.3, 47.7) centre (80.3, 47.7) ccw construction
  line L30 (79.3, 47.7) -> (79.3, 29.4) construction
  arc A7 (78.3, 28.4) -> (79.3, 29.4) centre (78.3, 29.4) ccw construction
  line L31 (78.3, 28.4) -> (70.7, 28.4) construction
  line L32 (70.7, 28.4) -> (70.7, 32.3) construction
  line L33 (70.7, 32.3) -> (68.7, 32.3) construction
  line L34 (68.7, 32.3) -> (68.7, 28.4) construction
  line L35 (68.7, 28.4) -> (48.7, 28.4) construction
  line L36 (48.7, 28.4) -> (48.7, 32.3) construction
  line L37 (48.7, 32.3) -> (46.7, 32.3) construction
  line L38 (46.7, 32.3) -> (46.7, 28.4) construction
  line L39 (46.7, 28.4) -> (32.9, 28.4) construction
  arc A8 (31.9, 29.4) -> (32.9, 28.4) centre (32.9, 29.4) ccw construction
  line L40 (31.9, 29.4) -> (31.9, 36.6) construction
  line L41 (31.9, 36.6) -> (13.058, 36.6) construction
  line L42 (13.058, 34.6) -> (15.058, 34.6) construction
  line L43 (15.058, 34.6) -> (15.058, 25) construction
  line L44 (15.058, 25) -> (20, 25) construction
  line L45 (20, 25) -> (20, 23) construction
  line L46 (20, 23) -> (22, 23) construction
  line L47 (22, 23) -> (22, 25) construction
  line L48 (22, 25) -> (27, 25) construction
  arc A9 (28, 24) -> (27, 25) centre (27, 24) ccw construction
  line L49 (28, 24) -> (28, -19) construction
  line L50 (28, -19) -> (26, -19) construction
  line L51 (26, -19) -> (26, -21) construction
  line L52 (26, -21) -> (28, -21) construction
  line L53 (26, -45.7) -> (26, -49.7) construction
  line L54 (28, -21) -> (28, -45.7) construction
  line L55 (28, -45.7) -> (26, -45.7) construction
  line L56 (26, -49.7) -> (28, -49.7) construction
  line L57 (28, -49.7) -> (28, -81.8) construction
  line L58 (28, -81.8) -> (26, -81.8) construction
  line L59 (26, -81.8) -> (26, -83.8) construction
  line L60 (26, -83.8) -> (28, -83.8) construction
  line L61 (28, -83.8) -> (28, -113.6) construction
  line L62 (28, -113.6) -> (26, -113.6) construction
  line L63 (26, -113.6) -> (26, -115.6) construction
  line L64 (26, -115.6) -> (28, -115.6) construction
  line L65 (28, -115.6) -> (28, -121.6) construction
  arc A10 (27, -122.6) -> (28, -121.6) centre (27, -121.6) ccw construction
  line L66 (27, -122.6) -> (1, -122.6) construction
  line L67 (1, -122.6) -> (1, -120.6) construction
  line L68 (1, -120.6) -> (-1, -120.6) construction
  line L69 (-1, -120.6) -> (-1, -122.6) construction
  line L70 (-1, -122.6) -> (-27, -122.6) construction
  arc A11 (-28, -121.6) -> (-27, -122.6) centre (-27, -121.6) ccw construction
  line L71 (-28, -121.6) -> (-28, -115.6) construction
  line L72 (-28, -115.6) -> (-26, -115.6) construction
  line L73 (-26, -115.6) -> (-26, -113.6) construction
  line L74 (-26, -113.6) -> (-28, -113.6) construction
  line L75 (-28, -113.6) -> (-28, -73.1) construction
  line L76 (-28, -73.1) -> (-26, -73.1) construction
  line L77 (-26, -73.1) -> (-26, -71.1) construction
  line L78 (-26, -71.1) -> (-28, -71.1) construction
  line L79 (-28, -71.1) -> (-28, -66.7) construction
  line L80 (-28, -66.7) -> (-35.3, -66.7) construction
  line L81 (-35.3, -66.7) -> (-35.3, -64.7) construction
  line L82 (-35.3, -64.7) -> (-37.3, -64.7) construction
  line L83 (-37.3, -64.7) -> (-37.3, -66.7) construction
  line L84 (-37.3, -66.7) -> (-58.048, -66.7) construction
  line L85 (-58.048, -66.7) -> (-58.048, -64.7) construction
  line L86 (-58.048, -64.7) -> (-60.048, -64.7) construction
  line L87 (-60.048, -64.7) -> (-60.048, -66.7) construction
  line L88 (-60.048, -66.7) -> (-66.048, -66.7) construction
  arc A12 (-67.048, -65.7) -> (-66.048, -66.7) centre (-66.048, -65.7) ccw construction
  line L89 (-67.048, -65.7) -> (-67.048, -57.2) construction
  arc A13 (-67.048, -57.2) -> (-71.048, -53.2) centre (-71.048, -57.2) ccw construction
  line L90 (-71.048, -53.2) -> (-78.3, -53.2) construction
  arc A14 (-79.3, -52.2) -> (-78.3, -53.2) centre (-78.3, -52.2) ccw construction
  line L91 (-79.3, -52.2) -> (-79.3, -29.7) construction
  arc A15 (-78.3, -28.7) -> (-79.3, -29.7) centre (-78.3, -29.7) ccw construction
  line L92 (-78.3, -28.7) -> (-72.3, -28.7) construction
  line L93 (-72.3, -28.7) -> (-72.3, -30.7) construction
  line L94 (-72.3, -30.7) -> (-70.3, -30.7) construction
  line L95 (-70.3, -30.7) -> (-70.3, -28.7) construction
  line L96 (-70.3, -28.7) -> (-37.3, -28.7) construction
  line L97 (-37.3, -28.7) -> (-37.3, -30.7) construction
  line L98 (-37.3, -30.7) -> (-35.3, -30.7) construction
  line L99 (-35.3, -30.7) -> (-35.3, -28.7) construction
  line L100 (-35.3, -28.7) -> (-28, -28.7) construction
  line L101 (-28, -28.7) -> (-28, -25.5) construction
  line L102 (-28, -25.5) -> (-26, -25.5) construction
  line L103 (-26, -25.5) -> (-26, -23.5) construction
  line L104 (-26, -23.5) -> (-28, -23.5) construction
  line L105 (-28, -23.5) -> (-28, 7.6) construction
  line L106 (-28, 7.6) -> (-26, 7.6) construction
  line L107 (-87.3, 69.858) -> (90.3, 69.858) construction
  line L108 (-87.3, -130.6) -> (-87.3, 69.858) construction
  line L109 (90.3, -130.6) -> (-87.3, -130.6) construction
  line L110 (90.3, 69.858) -> (90.3, -130.6) construction
  line L111 (-20.3, -28.5) -> (-20.3, -32.442) construction
  line L112 (-20.3, -32.442) -> (-18.3, -32.442) construction
  line L113 (-18.3, -32.442) -> (-18.3, -28.5) construction
  line L114 (-18.3, -28.5) -> (-20.3, -28.5) construction
  line L115 (-20.3, -62.958) -> (-20.3, -66.1) construction
  line L116 (-20.3, -66.1) -> (-18.3, -66.1) construction
  line L117 (-18.3, -66.1) -> (-18.3, -62.958) construction
  line L118 (-18.3, -62.958) -> (-20.3, -62.958) construction
  arc A16 (-73.3, -30.7) -> (-73.3, -28.7) centre (-73.3, -29.7) ccw
  arc A17 (-69.3, -28.7) -> (-69.3, -30.7) centre (-69.3, -29.7) ccw
  line L119 (-78.3, -28.7) -> (-72.3, -28.7) construction
  line L120 (-70.3, -30.7) -> (-70.3, -28.7) construction
  line L121 (-73.3, -30.7) -> (-69.3, -30.7)
  line L122 (-70.3, -28.7) -> (-37.3, -28.7) construction
  line L123 (-69.3, -28.7) -> (-73.3, -28.7)
  arc A18 (-38.3, -30.7) -> (-38.3, -28.7) centre (-38.3, -29.7) ccw
  arc A19 (-34.3, -28.7) -> (-34.3, -30.7) centre (-34.3, -29.7) ccw
  line L124 (-38.3, -30.7) -> (-34.3, -30.7)
  line L125 (-35.3, -28.7) -> (-28, -28.7) construction
  line L126 (-34.3, -28.7) -> (-38.3, -28.7)
  arc A20 (-26, -26.5) -> (-28, -26.5) centre (-27, -26.5) ccw
  arc A21 (-28, -22.5) -> (-26, -22.5) centre (-27, -22.5) ccw
  line L127 (-26, -22.5) -> (-26, -26.5)
  line L128 (-28, -23.5) -> (-28, 7.6) construction
  line L129 (-28, -22.5) -> (-28, -26.5)
  line L130 (-28, -28.7) -> (-28, -25.5) construction
  arc A22 (-28, 10.6) -> (-26, 10.6) centre (-27, 10.6) ccw
  arc A23 (-26, 6.6) -> (-28, 6.6) centre (-27, 6.6) ccw
  line L131 (-28, 7.6) -> (-26, 7.6) construction
  line L132 (-26, 10.6) -> (-26, 6.6)
  line L133 (-28, 27.342) -> (-28, 9.6) construction
  line L134 (-28, 10.6) -> (-28, 6.6)
  arc A24 (-29.742, 34.342) -> (-27.742, 34.342) centre (-28.742, 34.342) ccw
  arc A25 (-27.742, 30.342) -> (-29.742, 30.342) centre (-28.742, 30.342) ccw
  line L135 (-27.742, 34.342) -> (-27.742, 30.342)
  line L136 (-29.742, 34.342) -> (-29.742, 30.342)
  arc A26 (-27.742, 44.858) -> (-29.742, 44.858) centre (-28.742, 44.858) ccw
  arc A27 (-29.742, 48.858) -> (-27.742, 48.858) centre (-28.742, 48.858) ccw
  line L137 (-27.742, 48.858) -> (-27.742, 44.858)
  line L138 (-29.742, 60.858) -> (-29.742, 47.858) construction
  line L139 (-29.742, 48.858) -> (-29.742, 44.858)
  arc A28 (13.058, 59) -> (15.058, 59) centre (14.058, 59) ccw
  line L140 (13.058, 59) -> (13.058, 55)
  line L141 (13.058, 36.6) -> (13.058, 34.6) projected
  line L142 (15.058, 60.858) -> (15.058, 58) construction
  line L143 (15.058, 59) -> (15.058, 56)
  line L144 (15.058, 56) -> (14.058, 56)
  line L145 (13.058, 56) -> (31.9, 56) construction
  arc A29 (15.058, 33.6) -> (13.058, 33.6) centre (14.058, 33.6) ccw
  line L146 (13.058, 37.6) -> (13.058, 33.6)
  line L147 (15.058, 33.6) -> (15.058, 36.6)
  line L148 (15.058, 36.6) -> (14.058, 36.6)
  line L149 (31.9, 36.6) -> (13.058, 36.6) construction
  arc A30 (19, 23) -> (19, 25) centre (19, 24) ccw
  arc A31 (23, 25) -> (23, 23) centre (23, 24) ccw
  line L150 (22, 25) -> (27, 25) construction
  line L151 (15.058, 25) -> (20, 25) construction
  line L152 (20, 25) -> (20, 23) construction
  line L153 (23, 23) -> (19, 23)
  line L154 (23, 25) -> (19, 25)
  arc A32 (49.7, 60.8) -> (48.7, 59.8) centre (49.7, 59.8) ccw
  arc A33 (46.7, 59.8) -> (45.7, 60.8) centre (45.7, 59.8) ccw
  arc A34 (45.7, 56.9) -> (46.7, 57.9) centre (45.7, 57.9) ccw
  arc A35 (48.7, 57.9) -> (49.7, 56.9) centre (49.7, 57.9) ccw
  line L155 (49.7, 56.9) -> (45.7, 56.9)
  line L156 (45.7, 60.8) -> (49.7, 60.8)
  line L157 (48.7, 60.8) -> (68.7, 60.8) construction
  line L158 (46.7, 60.8) -> (46.7, 56.9) construction
  line L159 (46.7, 59.8) -> (46.7, 57.9)
  line L160 (48.7, 56.9) -> (48.7, 60.8) construction
  line L161 (48.7, 59.8) -> (48.7, 57.9)
  arc A36 (68.7, 59.8) -> (67.7, 60.8) centre (67.7, 59.8) ccw
  arc A37 (71.7, 60.8) -> (70.7, 59.8) centre (71.7, 59.8) ccw
  arc A38 (67.7, 56.9) -> (68.7, 57.9) centre (67.7, 57.9) ccw
  arc A39 (70.7, 57.9) -> (71.7, 56.9) centre (71.7, 57.9) ccw
  line L162 (71.7, 56.9) -> (67.7, 56.9)
  line L163 (67.7, 60.8) -> (71.7, 60.8)
  line L164 (70.7, 60.8) -> (81.3, 60.8) construction
  line L165 (70.7, 56.9) -> (70.7, 60.8) construction
  line L166 (70.7, 59.8) -> (70.7, 57.9)
  line L167 (68.7, 60.8) -> (68.7, 56.9) construction
  line L168 (68.7, 59.8) -> (68.7, 57.9)
  arc A40 (45.7, 28.4) -> (46.7, 29.4) centre (45.7, 29.4) ccw
  arc A41 (48.7, 29.4) -> (49.7, 28.4) centre (49.7, 29.4) ccw
  arc A42 (67.7, 28.4) -> (68.7, 29.4) centre (67.7, 29.4) ccw
  arc A43 (70.7, 29.4) -> (71.7, 28.4) centre (71.7, 29.4) ccw
  arc A44 (49.7, 32.3) -> (48.7, 31.3) centre (49.7, 31.3) ccw
  arc A45 (46.7, 31.3) -> (45.7, 32.3) centre (45.7, 31.3) ccw
  arc A46 (68.7, 31.3) -> (67.7, 32.3) centre (67.7, 31.3) ccw
  arc A47 (71.7, 32.3) -> (70.7, 31.3) centre (71.7, 31.3) ccw
  line L169 (45.7, 32.3) -> (49.7, 32.3)
  line L170 (67.7, 32.3) -> (71.7, 32.3)
  line L171 (68.7, 32.3) -> (68.7, 28.4) construction
  line L172 (70.7, 28.4) -> (70.7, 32.3) construction
  line L173 (78.3, 28.4) -> (70.7, 28.4) construction
  line L174 (71.7, 28.4) -> (67.7, 28.4)
  line L175 (68.7, 28.4) -> (48.7, 28.4) construction
  line L176 (70.7, 31.3) -> (70.7, 29.4)
  line L177 (68.7, 31.3) -> (68.7, 29.4)
  line L178 (48.7, 28.4) -> (48.7, 32.3) construction
  line L179 (48.7, 31.3) -> (48.7, 29.4)
  line L180 (46.7, 32.3) -> (46.7, 28.4) construction
  line L181 (46.7, 31.3) -> (46.7, 29.4)
  line L182 (49.7, 28.4) -> (45.7, 28.4)
  line L183 (46.7, 28.4) -> (32.9, 28.4) construction
  arc A48 (-61.048, -66.7) -> (-61.048, -64.7) centre (-61.048, -65.7) ccw
  arc A49 (-57.048, -64.7) -> (-57.048, -66.7) centre (-57.048, -65.7) ccw
  arc A50 (-38.3, -66.7) -> (-38.3, -64.7) centre (-38.3, -65.7) ccw
  arc A51 (-34.3, -64.7) -> (-34.3, -66.7) centre (-34.3, -65.7) ccw
  line L184 (-61.048, -64.7) -> (-57.048, -64.7)
  line L185 (-57.048, -66.7) -> (-61.048, -66.7)
  line L186 (-60.048, -66.7) -> (-66.048, -66.7) construction
  line L187 (-38.3, -64.7) -> (-34.3, -64.7)
  line L188 (-28, -66.7) -> (-35.3, -66.7) construction
  line L189 (-34.3, -66.7) -> (-38.3, -66.7)
  line L190 (-37.3, -66.7) -> (-58.048, -66.7) construction
  arc A52 (-28, -70.1) -> (-26, -70.1) centre (-27, -70.1) ccw
  arc A53 (-26, -74.1) -> (-28, -74.1) centre (-27, -74.1) ccw
  line L191 (-26, -70.1) -> (-26, -74.1)
  line L192 (-28, -70.1) -> (-28, -74.1)
  line L193 (-28, -113.6) -> (-28, -73.1) construction
  arc A54 (-17.3, -62.958) -> (-18.3, -63.958) centre (-17.3, -63.958) ccw
  arc A55 (-18.3, -65.1) -> (-17.3, -66.1) centre (-17.3, -65.1) ccw
  arc A56 (-20.3, -63.958) -> (-21.3, -62.958) centre (-21.3, -63.958) ccw
  arc A57 (-21.3, -66.1) -> (-20.3, -65.1) centre (-21.3, -65.1) ccw
  line L194 (-21.3, -62.958) -> (-17.3, -62.958)
  line L195 (-17.3, -66.1) -> (-21.3, -66.1)
  line L196 (-18.3, -63.958) -> (-18.3, -65.1)
  line L197 (-20.3, -62.958) -> (-20.3, -66.1) construction
  line L198 (-20.3, -63.958) -> (-20.3, -65.1)
  arc A58 (-17.3, -28.5) -> (-18.3, -29.5) centre (-17.3, -29.5) ccw
  arc A59 (-18.3, -31.442) -> (-17.3, -32.442) centre (-17.3, -31.442) ccw
  arc A60 (-20.3, -29.5) -> (-21.3, -28.5) centre (-21.3, -29.5) ccw
  arc A61 (-21.3, -32.442) -> (-20.3, -31.442) centre (-21.3, -31.442) ccw
  line L199 (-17.3, -28.5) -> (-21.3, -28.5)
  line L200 (-21.3, -32.442) -> (-17.3, -32.442)
  line L201 (-20.3, -29.5) -> (-20.3, -31.442)
  line L202 (-18.3, -31.442) -> (-18.3, -29.5)
  arc A62 (-28, -112.6) -> (-26, -112.6) centre (-27, -112.6) ccw
  arc A63 (-26, -116.6) -> (-28, -116.6) centre (-27, -116.6) ccw
  line L203 (-26, -112.6) -> (-26, -116.6)
  line L204 (-28, -112.6) -> (-28, -116.6)
  arc A64 (-2, -122.6) -> (-2, -120.6) centre (-2, -121.6) ccw
  arc A65 (2, -120.6) -> (2, -122.6) centre (2, -121.6) ccw
  line L205 (2, -122.6) -> (-2, -122.6)
  line L206 (-1, -122.6) -> (-27, -122.6) construction
  line L207 (2, -120.6) -> (-2, -120.6)
  arc A66 (26, -112.6) -> (28, -112.6) centre (27, -112.6) ccw
  arc A67 (28, -116.6) -> (26, -116.6) centre (27, -116.6) ccw
  line L208 (26, -112.6) -> (26, -116.6)
  line L209 (28, -83.8) -> (28, -113.6) construction
  line L210 (28, -112.6) -> (28, -116.6)
  arc A68 (28, -84.8) -> (26, -84.8) centre (27, -84.8) ccw
  arc A69 (26, -80.8) -> (28, -80.8) centre (27, -80.8) ccw
  arc A70 (26, -44.7) -> (28, -44.7) centre (27, -44.7) ccw
  arc A71 (28, -50.7) -> (26, -50.7) centre (27, -50.7) ccw
  arc A72 (28, -22) -> (26, -22) centre (27, -22) ccw
  arc A73 (26, -18) -> (28, -18) centre (27, -18) ccw
  line L211 (26, -18) -> (26, -22)
  line L212 (28, 24) -> (28, -19) construction
  line L213 (28, -18) -> (28, -22)
  line L214 (28, -45.7) -> (28, -21) construction
  line L215 (26, -44.7) -> (26, -50.7)
  line L216 (28, -44.7) -> (28, -50.7)
  line L217 (28, -81.8) -> (28, -49.7) construction
  line L218 (26, -80.8) -> (26, -84.8)
  line L219 (28, -80.8) -> (28, -84.8)
  line L220 (26, -21) -> (28, -21) projected
  line L221 (28, -21) -> (28, -45.7) projected
  line L222 (-28.742, 61.858) -> (-6.6, 61.858) construction
  line L223 (-6.6, 61.858) -> (-6.6, 59.858) construction
  line L224 (-6.6, 59.858) -> (-4.6, 59.858) construction
  line L225 (-4.6, 59.858) -> (-4.6, 61.858) construction
  line L226 (13.058, 58) -> (13.058, 56) projected
  arc A74 (-7.6, 59.858) -> (-7.6, 61.858) centre (-7.6, 60.858) ccw
  arc A75 (-3.6, 61.858) -> (-3.6, 59.858) centre (-3.6, 60.858) ccw
  line L227 (-3.6, 59.858) -> (-7.6, 59.858)
  line L228 (-28.742, 61.858) -> (-6.6, 61.858) construction
  line L229 (-4.6, 59.858) -> (-4.6, 61.858) construction
  line L230 (-6.6, 61.858) -> (-6.6, 59.858) construction
  line L231 (-3.6, 61.858) -> (-7.6, 61.858)
  line L232 (15.558, 53.4) -> (31.4, 53.4)
  arc A76 (15.058, 53.9) -> (15.558, 53.4) centre (15.558, 53.9) ccw
  arc A77 (31.4, 53.4) -> (31.9, 53.9) centre (31.4, 53.9) ccw
  line L233 (31.9, 56) -> (31.9, 53.9)
  line L234 (15.058, 55) -> (15.058, 53.9)
  line L235 (31.9, 56) -> (13.058, 56) construction
  line L236 (15.058, 56) -> (31.9, 56)
  arc A78 (15.058, 55) -> (13.058, 55) centre (14.058, 55) ccw
  line L237 (15.558, 38.4) -> (31.4, 38.4)
  arc A79 (31.9, 37.9) -> (31.4, 38.4) centre (31.4, 37.9) ccw
  arc A80 (15.558, 38.4) -> (15.058, 37.9) centre (15.558, 37.9) ccw
  line L238 (31.9, 36.6) -> (31.9, 37.9)
  arc A81 (13.058, 37.6) -> (15.058, 37.6) centre (14.058, 37.6) ccw
  line L239 (15.058, 37.6) -> (15.058, 37.9)
  line L240 (14.058, 36.6) -> (31.9, 36.6)
  point P0 (0, 0)
  point P1 (28, -41.5)
  dimension "d95" = 2
  dimension "d96" = 2
  dimension "d97" = 2
  dimension "d98" = 2
  dimension "d99" = 2
  dimension "d100" = 2
  dimension "d101" = 2
  dimension "d102" = 2
  dimension "d103" = 2
  dimension "d104" = 2
  dimension "d105" = 2
  dimension "d106" = 2
  dimension "d107" = 2
  dimension "d109" = 2
  dimension "d111" = 2
  dimension "d112" = 2
  dimension "d113" = 2
  dimension "d114" = 2
  dimension "d115" = 2
  dimension "d116" = 2
  dimension "d117" = 2
  dimension "d118" = 2
  dimension "d119" = 2
  dimension "d120" = 2
  dimension "d121" = 2
  dimension "d122" = 2
  dimension "d123" = 2
  dimension "d124" = 2
  dimension "d125" = 2
  dimension "d126" = 2
  dimension "d127" = 2
  dimension "d128" = 2
  dimension "d129" = 2
  dimension "d130" = 2
  dimension "d131" = 2
  dimension "d132" = 2
  dimension "d133" = 2
  dimension "d134" = 2
  dimension "d135" = 2
  dimension "d136" = 2
  dimension "d137" = 2
  dimension "d138" = 2
  dimension "d139" = 2
  dimension "d140" = 2
  dimension "d141" = 2
  dimension "d142" = 2
  dimension "d143" = 2
  dimension "d144" = 2
  dimension "d145" = 2
  dimension "d146" = 2
  dimension "d147" = 2
  dimension "d148" = 2
  dimension "d149" = 2
  dimension "d150" = 2
  dimension "d151" = 2
  dimension "d152" = 2
  dimension "d155" = 2
  dimension "d156" = 2
  dimension "d264" = 2
  dimension "d265" = 2
  dimension "d267" = 2.6
  dimension "d268" = 1
  dimension "d269" = 1
  dimension "d270" = 2
  constraints: 157 tangent, 145 end point, 136 point on circle, 89 point on line, 66 centre point, 14 horizontal, 14 vertical, 4 collinear, 4 perpendicular
  measures "d95" diameter of A16
  measures "d96" diameter of A17
  measures "d97" diameter of A18
  measures "d98" diameter of A19
  measures "d99" diameter of A20
  measures "d100" diameter of A21
  measures "d101" diameter of A22
  measures "d102" diameter of A23
  measures "d103" diameter of A24
  measures "d104" diameter of A25
  measures "d105" diameter of A26
  measures "d106" diameter of A27
  measures "d107" diameter of A28
  measures "d109" diameter of A29
  measures "d111" diameter of A30
  measures "d112" diameter of A31
  measures "d113" diameter of A32